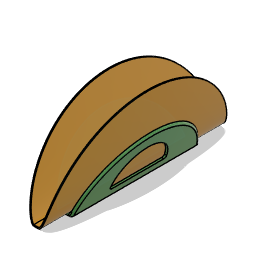
Taco Stand v2 (Autodesk Fusion 360 design; units mm, degrees)
Autodesk Fusion 360 part; units mm, degrees
sketch "Sketch1" plane through (0, 0, 0) normal (0, 0, 1) x (1, 0, 0) in component "Taco"
  line L0 (0, 0) -> (14, 0)
  line L1 (14, 0) -> (14, 58)
  line L2 (14, 58) -> (0, 58)
  line L3 (0, 58) -> (0, 0) construction
  spline S0 degree 5 poles (14, 58) (13.748357, 56.030394) (13.245896, 52.148548) (12.49468, 46.497873) (11.49809, 39.313546) (10.261462, 30.966643) (9.035222, 23.341956) (7.821127, 16.561841) (6.621274, 10.772081) (5.437747, 6.117593) (4.272244, 2.716328) (3.354522, 1.016173) (2.674206, 0.295666) (2.224154, 0.058103) (2, 0) knots 0 0 0 0 0 0 0.1 0.2 0.3 0.4 0.5 0.6 0.7 0.8 0.9 1 1 1 1 1 1
  line L4 (-14, 58) -> (0, 58)
  line L5 (-14, 0) -> (-14, 58)
  spline S1 degree 5 poles (-14, 58) (-13.748357, 56.030394) (-13.245896, 52.148548) (-12.49468, 46.497873) (-11.49809, 39.313546) (-10.261462, 30.966643) (-9.035222, 23.341956) (-7.821127, 16.561841) (-6.621274, 10.772081) (-5.437747, 6.117593) (-4.272244, 2.716328) (-3.354522, 1.016173) (-2.674206, 0.295666) (-2.224154, 0.058103) (-2, 0) knots 0 0 0 0 0 0 0.1 0.2 0.3 0.4 0.5 0.6 0.7 0.8 0.9 1 1 1 1 1 1
  line L6 (15.060168, 66.297924) -> (12.939832, 49.702076)
  line L7 (4.707721, 0.701875) -> (-0.707721, -0.701875)
  line L8 (-15.060168, 66.297924) -> (-12.939832, 49.702076)
  line L9 (-4.707721, 0.701875) -> (0.707721, -0.701875)
  line L10 (0, 0) -> (-14, 0)
  point P0 (2, 0)
  point P1 (5, 5)
  point P2 (-5, 5)
  dimension "d3" = 14
  dimension "d4" = 58
  constraint horizontal L0
  constraint vertical L1
  constraint horizontal L2
  constraint vertical L3
  constraint coincident L0.start L3.end
  constraint coincident L0 P0
  constraint coincident P0 S0.end
  constraint midpoint L1.end L6
  constraint midpoint P0 L7
  constraint symmetric L0.start L3 L10.start
  constraint symmetric L0.end L3 L5.start
  constraint symmetric L1.end L3 L4.start
  constraint symmetric L2.end L3 L4.end
  constraint symmetric L3 P1 P2
  constraint symmetric L3 P0 S1.end
  measures "d3" distance of L0.start L0.end
  measures "d4" distance of L0.start L2.end
extrude "Extrude1" add sketch "Sketch1" along normal mid plane 130 contours L0 L2 S0 L4 S1 L10 picked at (0, 32.961993) makes body 1 in component "Taco"
sketch "Sketch2" plane through (0, 0, 0) normal (1, 0, 0) x (0, 0, -1) in component "Taco"
  line L0 (65, 58) -> (-65, 58)
  line L1 (-65, 0) -> (-65, 58)
  line L2 (-65, 0) -> (65, 0)
  line L3 (65, 58) -> (65, 0)
  arc A0 (65, 0) -> (-65, 0) centre (0, -7.422414) ccw
  constraint tangent L0 A0
  constraint coincident L2.end L3.end
  constraint coincident L1.start L2.start
extrude "Extrude2" cut sketch "Sketch2" along normal mid plane 30 contours L0 L3 A0 | L0 L1 A0 picked at (52.913627, 44.647437) picked at (-52.913627, 44.647437) bodies 1 in component "Taco"
shell "Shell1" thickness 0.8 removed faces 1 at (-4.409539, 54.014458, 22.485617) on bodies 1 in component "Taco"
sketch "Sketch1 (2)" plane through (0, 0, 0) normal (0, 0, 1) x (1, 0, 0) in component "Taco Stand"
  line L0 (0, 0) -> (-3.71658, 0)
  line L1 (-3.71658, 0) -> (-16.024201, 33.814912)
  line L2 (0, -1.5) -> (-4.766891, -1.5)
  line L3 (-4.766891, -1.5) -> (-17.43374, 33.301882)
  line L4 (-16.024201, 33.814912) -> (-17.43374, 33.301882)
  line L5 (0, 39.000001) -> (0, -11) construction
  line L6 (3.71658, 0) -> (16.024201, 33.814912)
  line L7 (16.024201, 33.814912) -> (17.43374, 33.301882)
  line L8 (4.766891, -1.5) -> (17.43374, 33.301882)
  line L9 (0, 0) -> (3.71658, 0)
  line L10 (0, -1.5) -> (4.766891, -1.5)
  dimension "d10" = -1.5
  dimension "d11" = 110
  constraint coincident L0.start L9.start
  constraint horizontal L0
  constraint vertical L5
  constraint symmetric L0.start L5 L9.start
  constraint symmetric L2.start L5 L10.start
  measures "d11" angle of L0 L1
sketch "Sketch2 (2)" plane through (0, 0, 0) normal (0, 0, 1) x (1, 0, 0) in component "Taco Stand"
extrude "Extrude1'" add sketch "Sketch1 (2)" along normal mid plane 90 separate body makes body 2 in component "Taco Stand"
sketch "Sketch3" plane through (4.691361, -1.707516, 0) normal (0.939693, -0.34202, 0) x (0, 0, -1) in component "Taco Stand"
  line L0 (45, 37.256223) -> (-45, 37.256223)
  line L1 (-45, 37.256223) -> (-45, 0.220834)
  line L2 (-45, 0.220834) -> (45, 0.220834)
  line L3 (45, 0.220834) -> (45, 37.256223)
  arc A0 (45, 0.220834) -> (-45, 0.220834) centre (0, -8.600188) ccw
  constraint tangent L0 A0
extrude "Extrude2'" cut sketch "Sketch3" against normal blind 2 contours L0 L3 A0 | L0 L1 A0 picked at (35.955185, 28.844658) picked at (-35.955185, 28.844658) bodies 2 in component "Taco Stand"
sketch "Sketch4" plane through (-4.691361, -1.707516, 0) normal (-0.939693, -0.34202, 0) x (0, 0, 1) in component "Taco Stand"
  line L0 (-45, 0.220834) -> (45, 0.220834)
  line L1 (45, 0.220834) -> (45, 37.256223)
  line L2 (45, 37.256223) -> (-45, 37.256223)
  line L3 (-45, 37.256223) -> (-45, 0.220834)
  arc A0 (45, 0.220834) -> (-45, 0.220834) centre (0, -8.600188) ccw
  constraint tangent L2 A0
extrude "Extrude3" cut sketch "Sketch4" against normal blind 2 contours L2 L3 A0 | L1 L2 A0 picked at (-35.955185, 28.844658) picked at (35.955185, 28.844658) bodies 2 in component "Taco Stand"
sketch "Sketch5" plane through (-4.691361, -1.707516, 0) normal (-0.939693, -0.34202, 0) x (0, 0, 1) in component "Taco Stand"
  arc A0 (45, 0.220834) -> (-45, 0.220834) centre (0, -8.600188) ccw
  line L0 (-45, 0.220834) -> (45, 0.220834)
ref_plane "WorkPlane1" through (0, 18.647872, 0) normal (1, 0, 0) x (0, 1, 0) in component "Taco Stand"
sketch "Sketch6" plane through (0, 18.647872, 0) normal (1, 0, 0) x (0, 0, -1) in component "Taco Stand"
  line L0 (-20, -15) -> (20, -15)
  line L1 (20, -15) -> (20, 5)
  line L2 (20, 5) -> (-20, 5)
  line L3 (-20, 5) -> (-20, -15)
  line L4 (-20, -15) -> (20, 5) construction
  line L5 (20, -15) -> (-20, 5) construction
  arc A0 (20, -15) -> (-20, -15) centre (0, -15) ccw
  point P0 (0, -5)
  constraint horizontal L0
  constraint perpendicular L0 L1
  constraint parallel L0 L2
  constraint parallel L1 L3
  constraint coincident L4 P0
  constraint coincident L5 P0
  constraint tangent L2 A0
extrude "Extrude4" cut sketch "Sketch6" along normal through all and the other way through all contours L0 A0 picked at (-2.577102, -4.035452) bodies 2 in component "Taco Stand"
fillet "Fillet1" radius 1.5 2 edges at (3.71658, 0, 0) (-3.71658, 0, 0) on bodies 2 in component "Taco Stand"
fillet "Fillet2" radius 1.5 4 edges at (-5.84243, 3.647872, 20) (5.84243, 3.647872, 20) (5.84243, 3.647872, -20) (-5.84243, 3.647872, -20) on bodies 2 in component "Taco Stand"
fillet "Fillet3" radius 1.5 6 edges at (-2.950044, 0.027087, -45) (0, 0, -45) (2.950044, 0.027087, -45) (2.950044, 0.027087, 45) (0, 0, 45) (-2.950044, 0.027087, 45) on bodies 2 in component "Taco Stand"
fillet "Fillet4" radius 1.5 1 edges at (17.43374, 33.301882, 0) on bodies 2 in component "Taco Stand"
fillet "Fillet5" radius 1.5 1 edges at (-17.43374, 33.301882, 0) on bodies 2 in component "Taco Stand"
component "Taco" placed x (1, 0, 0) y (0, 1, 0) z (0, 0, 1) at (0, 0, 0)
component "Taco Stand" placed x (1, 0, 0) y (0, 1, 0) z (0, 0, 1) at (0, 0, 0)
